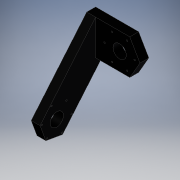
# Autodesk Inventor part: HA07
Saved by Autodesk Inventor 2017 (Build 210142000, 142)
## iProperties
Created: 2018-11-27
Part Number: HA07
Material: ABS Plastic
Document SubType Name: Modeling
Designer: Dell
Density: 1.06 g/cm^3
Appearance: Smooth - Black
Author: Dell
Autodesk Inventor part; units mm, degrees
ref_plane "YZ Plane" through (0, 0, 0) normal (1, 0, 0) x (0, 1, 0)
ref_plane "XZ Plane" through (0, 0, 0) normal (0, 1, 0) x (-1, 0, 0)
ref_plane "XY Plane" through (0, 0, 0) normal (0, 0, 1) x (1, 0, 0)
sketch "Sketch1" plane through (0, 0, 0) normal (0, 0, 1) x (1, 0, 0)
  line L0 (51, 0) -> (25.5, -44.1673) construction
  line L1 (25.5, -44.1673) -> (-25.5, -44.1673) construction
  line L2 (-25.5, -44.1673) -> (-51, 0) construction
  line L3 (-51, 0) -> (-25.5, 44.1673) construction
  line L4 (-25.5, 44.1673) -> (25.5, 44.1673) construction
  line L5 (25.5, 44.1673) -> (51, 0) construction
  circle A0 centre (51, 0) radius 2.5
  circle A1 centre (0, 0) radius 22.5
  circle A2 centre (25.5, 44.1673) radius 2.5
  circle A3 centre (-25.5, 44.1673) radius 2.5
  circle A4 centre (-51, 0) radius 2.5
  circle A5 centre (-25.5, -44.1673) radius 2.5
  circle A6 centre (25.5, -44.1673) radius 2.5
  line L6 (57.5, 0) -> (28.75, -49.7965)
  line L7 (28.75, -49.7965) -> (-28.75, -49.7965)
  line L8 (-28.75, -49.7965) -> (-57.5, 0)
  line L9 (-57.5, 0) -> (-28.75, 49.7965)
  line L10 (-28.75, 49.7965) -> (28.75, 49.7965)
  line L11 (28.75, 49.7965) -> (57.5, 0)
  dimension "d0" = 102
  dimension "d1" = 5
  dimension "d2" = 45
  dimension "d5" = 360
  dimension "d7" = 115
  constraints: 24 end point, 7 centre point, 4 coincident, 2 horizontal alignment, 39 other
  measures "d0" distance of L0.start L2.end
  measures "d1" diameter of A0
  measures "d2" diameter of A1
  measures "d7" distance of L6.start L8.end
extrude "Extrusion1" add sketch "Sketch1" along normal blind 30
sketch "Sketch6" plane through (0, 0, 30) normal (0, 0, 1) x (1, 0, 0)
  line L0 (28.75, 49.7965) -> (-28.75, 49.7965) projected
  line L1 (-28.75, 49.7965) -> (-111.25, 49.7965)
  line L2 (-111.25, 49.7965) -> (-111.25, -49.7965)
  line L3 (-111.25, -49.7965) -> (-28.75, -49.7965)
  line L4 (-28.75, 49.7965) -> (-57.5, 0) projected
  line L5 (-57.5, 0) -> (-28.75, -49.7965) projected
  point P0 (0, 0)
  dimension "d68" = 111.25
  constraints: 6 end point, 2 perpendicular, 1 horizontal
  measures "d68" distance from line of point (0, 0) L2
extrude "Extrusion6" add sketch "Sketch6" against normal blind 30
sketch "Sketch7" plane through (-111.25, -49.7965, 30) normal (-1, 0, 0) x (0, 0, 1)
  line L0 (0, 99.5929) -> (0, 0) projected
  line L1 (0, 99.5929) -> (-30, 99.5929) projected
  line L2 (-30, 0) -> (-30, 99.5929) projected
  line L3 (0, 0) -> (-30, 0) projected
  line L4 (151.0551, -70.6307) -> (188.0154, -114.6783)
  line L5 (188.0154, -114.6783) -> (168.3492, -168.7106)
  line L6 (168.3492, -168.7106) -> (111.7228, -178.6954)
  line L7 (111.7228, -178.6954) -> (74.7625, -134.6478)
  line L8 (74.7625, -134.6478) -> (94.4286, -80.6155)
  line L9 (94.4286, -80.6155) -> (151.0551, -70.6307)
  line L10 (74.7625, -134.6478) -> (188.0154, -114.6783)
  line L11 (-30, -9.7968) -> (74.7625, -134.6478)
  line L12 (-30, -9.7968) -> (-30, 109.3897)
  line L13 (-30, 109.3897) -> (0, 109.3897)
  line L14 (0, 109.3897) -> (151.0551, -70.6307)
  point P0 (131.3889, -124.6631)
  point P1 (-30, 49.7965)
  dimension "d43" = 115
  dimension "d48" = 40
  dimension "d49" = 235
  constraints: 22 end point, 2 collinear, 2 midpoint, 1 perpendicular, 1 vertical, 1 vertical alignment, 13 other
  measures "d43" distance of L7.end L4.end
  measures "d48" angle of L14 L0
  measures "d49" distance of L13.end L4.start
extrude "Extrusion7" add sketch "Sketch7" against normal blind 30
sketch "Sketch8" plane through (0, 0, 0) normal (0, 0, -1) x (-1, 0, 0)
  line L0 (-68.8123, 0) -> (-34.4062, 59.5932)
  line L1 (-34.4062, 59.5932) -> (34.4062, 59.5932)
  line L2 (34.4062, 59.5932) -> (68.8123, 0)
  line L3 (68.8123, 0) -> (34.4062, -59.5932)
  line L4 (34.4062, -59.5932) -> (-34.4062, -59.5932)
  line L5 (-34.4062, -59.5932) -> (-68.8123, 0)
  line L6 (111.25, 59.5932) -> (81.25, 59.5932) projected
  line L7 (81.25, 59.5932) -> (34.4062, 59.5932)
  line L8 (81.25, -59.5932) -> (34.4062, -59.5932)
  line L9 (111.25, -59.5932) -> (81.25, -59.5932) projected
  line L10 (81.25, 49.7965) -> (-28.75, 49.7965) projected
  line L11 (-28.75, 49.7965) -> (-57.5, 0) projected
  line L12 (-57.5, 0) -> (-28.75, -49.7965) projected
  line L13 (-28.75, -49.7965) -> (81.25, -49.7965) projected
  line L14 (81.25, -59.5932) -> (81.25, -49.7965) projected
  line L15 (111.25, -59.5932) -> (81.25, -59.5932) projected
  line L16 (111.25, 59.5932) -> (111.25, -59.5932) projected
  line L17 (111.25, 59.5932) -> (81.25, 59.5932) projected
  line L18 (81.25, 49.7965) -> (81.25, 59.5932) projected
  circle A0 centre (-51, 0) radius 2.5 projected
  circle A1 centre (-25.5, 44.1673) radius 2.5 projected
  circle A2 centre (25.5, 44.1673) radius 2.5 projected
  circle A3 centre (51, 0) radius 2.5 projected
  circle A4 centre (25.5, -44.1673) radius 2.5 projected
  circle A5 centre (-25.5, -44.1673) radius 2.5 projected
  circle A6 centre (0, 0) radius 22.5 projected
  line L19 (81.25, 49.7965) -> (-28.75, 49.7965) projected
  line L20 (40.0623, 49.7965) -> (-28.75, 49.7965)
  line L21 (-28.75, 49.7965) -> (-57.5, 0)
  line L22 (-28.75, -49.7965) -> (-57.5, 0) projected
  line L23 (-28.75, -49.7965) -> (-57.5, 0)
  line L24 (-28.75, -49.7965) -> (40.0623, -49.7965)
  line L25 (-28.75, -49.7965) -> (81.25, -49.7965) projected
  line L26 (34.4062, 59.5932) -> (81.25, 59.5932)
  line L27 (81.25, 59.5932) -> (81.25, -164.4748) projected
  line L28 (81.25, 49.7965) -> (81.25, 59.5932)
  line L29 (40.0623, 49.7965) -> (81.25, 49.7965)
  line L30 (40.0623, -49.7965) -> (81.25, -49.7965)
  line L31 (81.25, -228.4919) -> (81.25, -59.5932) projected
  line L32 (81.25, -49.7965) -> (81.25, -59.5932)
  line L33 (81.25, -59.5932) -> (34.4062, -59.5932)
  constraints: 36 end point, 6 collinear, 4 point on line, 2 parallel, 1 coincident, 1 perpendicular, 1 vertical, 13 other
extrude "Extrusion8" add sketch "Sketch8" against normal blind 30 contours L0 L1 L2 L10 L11 L12 L13 L3 L4 L5 | L7 L18 L10 L2 | L3 L13 L14 L8
sketch "Sketch9" plane through (-111.25, -228.4919, 141.7228) normal (-1, 0, 0) x (0, 0.1736482, 0.9848078)
  line L0 (57.5, 0) -> (86.25, 49.7965) construction
  line L1 (0, 0) -> (57.5, 0) construction
  line L2 (57.5, 0) -> (0, 0)
  line L3 (0, 0) -> (-28.75, 49.7965) construction
  line L4 (-28.75, 49.7965) -> (0, 99.5929) construction
  line L5 (0, 99.5929) -> (57.5, 99.5929) construction
  line L6 (57.5, 99.5929) -> (86.25, 49.7965) construction
  line L7 (86.25, 49.7965) -> (57.5, 0)
  circle A0 centre (3.25, 93.9638) radius 2.5
  line L8 (0, 99.5929) -> (28.75, 49.7965) construction
  circle A1 centre (28.75, 49.7965) radius 22.5
  circle A2 centre (-22.25, 49.7965) radius 2.5
  circle A3 centre (3.25, 5.6292) radius 2.5
  circle A4 centre (54.25, 5.6292) radius 2.5
  circle A5 centre (79.75, 49.7965) radius 2.5
  circle A6 centre (54.25, 93.9638) radius 2.5
  point P0 (-99.8925, 249.6305)
  dimension "d52" = 5
  dimension "d53" = 45
  dimension "d55" = 51
  dimension "d58" = 360
  constraints: 14 end point, 7 centre point, 1 coincident, 1 point on line, 26 other
  measures "d52" diameter of A0
  measures "d53" diameter of A1
  measures "d55" distance of L8.end A0.centre
extrude "Extrusion9" cut sketch "Sketch9" against normal through all
body "Solid1"
